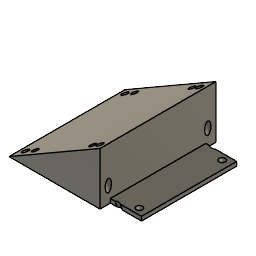
雷达30° (Autodesk Fusion 360 design; units mm, degrees)
part number: 2026-06-11-09-27-46-250
Autodesk Fusion 360 part; units mm, degrees
note: some values were not read from the file. Set by a fixed rule: which sketch regions a step uses.
sketch "草图1" plane through (0, 0, 0) normal (0, 0, 1) x (1, 0, 0)
  line L0 (18, 24) -> (-18, 24)
  line L1 (-18, 24) -> (-18, -24)
  line L2 (-18, -24) -> (18, -24)
  line L3 (18, -24) -> (18, 24)
  line L4 (18, 24) -> (-18, -24) construction
  line L5 (-18, 24) -> (18, -24) construction
  circle A0 centre (18, 24) radius 1.5
  circle A1 centre (-18, 24) radius 1.5
  circle A2 centre (-18, -24) radius 1.5
  circle A3 centre (18, -24) radius 1.5
  line L6 (22, 28) -> (-22, 28)
  line L7 (-22, 28) -> (-22, -28)
  line L8 (-22, -28) -> (22, -28)
  line L9 (22, -28) -> (22, 28)
  line L10 (22, 28) -> (-22, -28) construction
  line L11 (-22, 28) -> (22, -28) construction
  dimension "d1" = 36
  dimension "d2" = 48
  dimension "d3" = 3
  dimension "d4" = 3
  dimension "d5" = 3
  dimension "d6" = 3
  constraint horizontal L0
  constraint perpendicular L0 L1
  constraint parallel L0 L2
  constraint parallel L1 L3
  constraint coincident L4 origin
  constraint coincident L5 origin
  constraint coincident L0.start L3.end
  constraint coincident L0.end L1.start
  constraint coincident L1.end L2.start
  constraint coincident L2.end L3.start
  constraint horizontal L6
  constraint perpendicular L6 L7
  constraint parallel L6 L8
  constraint parallel L7 L9
  constraint coincident L10 origin
  constraint coincident L11 origin
  measures "d1" distance of L1.end L2.end
  measures "d2" distance of L0.end L1.end
  measures "d3" diameter of A0
  measures "d4" diameter of A1
  measures "d5" diameter of A2
  measures "d6" diameter of A3
extrude "拉伸1" add sketch "草图1" along normal blind 20 contours L0 L1 L2 L3 A0 A1 A2 A3 | L6 L7 L8 L9
sketch "草图2" plane through (0, -28, 0) normal (0, -1, 0) x (1, 0, 0)
  line L0 (-22, 0) -> (22, 0)
  line L1 (22, 0) -> (22, 20)
  line L2 (22, 20) -> (-22, 20)
  line L3 (-22, 20) -> (-22, 0)
  line L4 (-22, 0) -> (22, 25.4034)
  line L5 (-22, 0) -> (29.1908, 0) construction
  line L6 (22, 0) -> (22, 25.4034)
  line L7 (-22, 0) -> (22, 25.4034)
  line L8 (22, 25.4034) -> (22, 46)
  line L9 (22, 46) -> (-23, 46)
  line L10 (-23, 46) -> (-22, 0)
  dimension "d9" = 30
  constraint horizontal L5
  constraint coincident L0.start L3.end
  constraint coincident L0.end L1.start
  constraint coincident L4 L6.end
  constraint perpendicular L0 L6
  constraint parallel L4 L7
  constraint perpendicular L0 L8
  constraint perpendicular L8 L9
  measures "d9" angle of L4 L5
extrude "拉伸2" add sketch "草图2" against normal blind 56 contours L2 L4 L6 L7
extrude "拉伸3" cut sketch "草图2" against normal blind 74 contours L2 L3 L4 L7
extrude "拉伸4" cut 1 faces at (18.1827, -24.4654, 20) along direction (0, 0, 1) blind 10
extrude "拉伸5" cut 1 faces at (18.8158, 24.2169, 20) along direction (0, 0, 1) blind 10
sketch "草图3" plane through (0, 0, 0) normal (0, 0, -1) x (1, 0, 0)
  circle A0 centre (18, -24) radius 1.5
  circle A1 centre (18, 24) radius 1.5
  circle A2 centre (-18, 24) radius 1.5
  circle A3 centre (-18, -24) radius 1.5
  line L0 (22, -28) -> (22, 28)
  line L1 (22, 28) -> (-22, 28)
  line L2 (-22, 28) -> (-22, -28)
  line L3 (-22, -28) -> (22, -28)
extrude "拉伸6" add sketch "草图3" against normal blind 21 contours A0 | A1 | A2 | A3
sketch "草图4" plane through (0, 0, 21) normal (0, 0, 1) x (-1, 0, 0)
  circle A0 centre (-18, 24) radius 1.5
extrude "拉伸7" add sketch "草图4" 1 faces at (17.6113, 22.9591, 21) along normal blind 20
extrude "拉伸8" cut sketch "草图2" against normal blind 75 contours L2 L3 L4 L7 L8 L9 L10 | L2 L3 L4 L7
sketch "草图5" plane through (-5.5, 0, 9.5263) normal (-0.5, 0, 0.866025) x (0, -1, 0)
  line L0 (28, -19.0526) -> (28, 31.7543)
  line L1 (28, 31.7543) -> (-28, 31.7543)
  line L2 (-28, 31.7543) -> (-28, -19.0526)
  line L3 (-28, -19.0526) -> (28, -19.0526)
  line L4 (24, 23) -> (-24, 23)
  line L5 (-24, 23) -> (-24, -9)
  line L6 (-24, -9) -> (24, -9)
  line L7 (24, -9) -> (24, 23)
  line L8 (24, 23) -> (-24, -9) construction
  line L9 (-24, 23) -> (24, -9) construction
  circle A0 centre (-24, 23) radius 1.5
  circle A1 centre (-24, -9) radius 1.5
  circle A2 centre (24, -9) radius 1.5
  circle A3 centre (24, 23) radius 1.5
  point P0 (0, 7)
  dimension "d24" = 48
  dimension "d25" = 32
  dimension "d26" = 3
  dimension "d27" = 3
  dimension "d28" = 3
  dimension "d29" = 3
  constraint horizontal L4
  constraint perpendicular L4 L5
  constraint parallel L4 L6
  constraint parallel L5 L7
  constraint coincident L8 P0
  constraint coincident L9 P0
  constraint coincident L4.end L5.start
  constraint coincident L5.end L6.start
  constraint coincident L6.end L7.start
  constraint coincident L4.start L7.end
  measures "d24" distance of L5.end L6.end
  measures "d25" distance of L4.end L5.end
  measures "d26" diameter of A0
  measures "d27" diameter of A1
  measures "d28" diameter of A2
  measures "d29" diameter of A3
extrude "拉伸9" cut sketch "草图5" against normal blind 52 contours L4 L5 A0 | L4 L5 A0 | L4 L7 A3 | L4 L7 A3 | L5 L6 A1 | L5 L6 A1 | L6 L7 A2 | L6 L7 A2
sketch "草图6" plane through (0, -28, 0) normal (0, -1, 0) x (1, 0, 0)
  line L0 (22, 25.4034) -> (-22, 0)
  line L1 (-22, 0) -> (22, 0)
  line L2 (22, 0) -> (22, 25.4034)
  line L3 (19, 3) -> (-10, 3)
  line L4 (-10, 3) -> (19, 19.7432)
  line L5 (19, 19.7432) -> (19, 3)
  dimension "d32" = 30
  constraint perpendicular L2 L3
  constraint perpendicular L3 L5
  measures "d32" angle of L3 L4
extrude "拉伸10" cut sketch "草图6" against normal blind 100 contours L3 L4 L5
sketch "草图7" plane through (0, 0, 0) normal (0, 0, -1) x (1, 0, 0)
  ellipse E0 centre (-10.3923, 24) end of major axis (-12.1244, 24) minor radius 1.5
  ellipse E1 centre (-10.3923, -24) end of major axis (-12.1244, -24) minor radius 1.5
  line L0 (22, -28) -> (22, 28)
  line L1 (22, 28) -> (-22, 28)
  line L2 (-22, 28) -> (-22, -28)
  line L3 (-22, -28) -> (22, -28)
  line L4 (-17, 0) -> (-17, 15)
  line L5 (-17, 15) -> (-17, -15)
  circle A0 centre (-17, -15) radius 1.5
  circle A1 centre (-17, 15) radius 1.5
  line L6 (-17, 0) -> (33, 0)
  line L7 (33, 0) -> (33, 20)
  line L8 (33, 20) -> (33, -20)
  dimension "d35" = 3
  dimension "d36" = 3
  constraint parallel L2 L4
  constraint parallel L2 L5
  constraint coincident L5.end A0.centre
  constraint coincident L4.end L5.start
  constraint perpendicular L4 L6
  constraint perpendicular L6 L7
  constraint parallel L7 L8
  measures "d35" diameter of A0
  measures "d36" diameter of A1
sketch "草图8" plane through (22, 0, 0) normal (1, 0, 0) x (0, 1, 0)
  ellipse E0 centre (-24, 7.8949) end of major axis (-24, 4.8949) minor radius 1.5
  ellipse E1 centre (24, 7.8949) end of major axis (24, 4.8949) minor radius 1.5
  line L0 (-28, 0) -> (28, 0)
  line L1 (28, 0) -> (28, 25.4034)
  line L2 (28, 25.4034) -> (-28, 25.4034)
  line L3 (-28, 25.4034) -> (-28, 0)
  line L4 (-22, 0) -> (-22, 2)
  line L5 (-22, 2) -> (22, 2)
  line L6 (22, 2) -> (22, 0)
  constraint coincident L0 L4.start
  constraint perpendicular L0 L4
  constraint perpendicular L4 L5
  constraint coincident L0 L6.end
  constraint perpendicular L0 L6
extrude "拉伸11" add sketch "草图8" along normal blind 15 contours L0 L4 L5 L6
sketch "草图9" plane through (0, 0, 0) normal (0, 0, -1) x (1, 0, 0)
  ellipse E0 centre (-10.3923, 24) end of major axis (-12.1244, 24) minor radius 1.5
  ellipse E1 centre (-10.3923, -24) end of major axis (-12.1244, -24) minor radius 1.5
  line L0 (22, 22) -> (22, 28)
  line L1 (22, 28) -> (-22, 28)
  line L2 (-22, 28) -> (-22, -28)
  line L3 (-22, -28) -> (22, -28)
  line L4 (22, -28) -> (22, -22)
  line L5 (22, -22) -> (37, -22)
  line L6 (37, -22) -> (37, 22)
  line L7 (37, 22) -> (22, 22)
  circle A0 centre (33, -20) radius 1.5
  circle A1 centre (33, 20) radius 1.5
  dimension "d39" = 3
  dimension "d40" = 3
  measures "d39" diameter of A0
  measures "d40" diameter of A1
extrude "拉伸12" add 1 faces at (27, -22, 0.6667) along direction (0, -1, 0) blind 1
extrude "拉伸13" add 1 faces at (27, 22, 1.3333) along direction (0, 1, 0) blind 1
extrude "拉伸14" cut sketch "草图7" sketch "草图9" against normal blind 133 contours A0 | A1 of sketch 2 contours A0 | A1
sketch "草图10" plane through (0, -28, 0) normal (0, -1, 0) x (1, 0, 0)
  line L0 (19, 3) -> (-10, 3)
  line L1 (-10, 3) -> (19, 19.7432)
  line L2 (19, 19.7432) -> (19, 3)
  line L3 (22, 25.4034) -> (-22, 0)
  line L4 (-22, 0) -> (22, 0)
  line L5 (22, 0) -> (22, 25.4034)
  line L6 (22, 25.4034) -> (22, 0)
  line L7 (-22, 0) -> (22, 0)
  line L8 (22, 25.4034) -> (-22, 0)
  constraint coincident L3.start L5.end
  constraint coincident L4.end L5.start
  constraint coincident L3.end L4.start
extrude "拉伸15" add sketch "草图10" against normal blind 56 contours L0 L1 L2 | L3 L4 L5 L6 L7 L8
extrude "拉伸16" cut sketch "草图5" against normal blind 100 contours L4 L5 A0 | L4 L5 A0 | L4 L7 A3 | L4 L7 A3 | L5 L6 A1 | L5 L6 A1 | L6 L7 A2 | L6 L7 A2
extrude "拉伸17" add sketch "草图1" against normal blind 100 contours L0 L1 A1 | L0 L1 A1 | L0 L3 A0 | L0 L3 A0 | L1 L2 A2 | L1 L2 A2 | L2 L3 A3 | L2 L3 A3
extrude "拉伸18" cut 4 faces at (-18.3887, -22.9591, -100) (17.6113, -22.9591, -100) (17.6113, 25.0409, -100) (-18.3887, 25.0409, -100) along direction (0, 0, 1) blind 200
